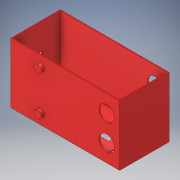
# Autodesk Inventor part: Torse
Saved by Autodesk Inventor 2019 (Build 230136000, 136)
## iProperties
Created: 2020-01-16
Part Number: Torse
Material: Générique
Document SubType Name: Modeling
Designer: Quentin
Density: 1 g/cm^3
Appearance: Rouge clair
Author: Quentin
Autodesk Inventor part; units mm, degrees
ref_plane "YZ Plane" through (0, 0, 0) normal (1, 0, 0) x (0, 1, 0)
ref_plane "XZ Plane" through (0, 0, 0) normal (0, 1, 0) x (-1, 0, 0)
ref_plane "XY Plane" through (0, 0, 0) normal (0, 0, 1) x (1, 0, 0)
sketch "Esquisse1" plane through (0, 0, 0) normal (1, 0, 0) x (0, 1, 0)
  line L0 (0, 0) -> (60, 0)
  line L1 (60, 0) -> (60, -50)
  line L2 (60, -50) -> (0, -50)
  line L3 (0, -50) -> (0, 0)
  dimension "d0" = 60
  dimension "d1" = 50
  constraints: 8 end point, 2 parallel, 1 horizontal, 1 perpendicular
  measures "d0" distance of L1.end L2.end
  measures "d1" distance of L0.end L1.end
extrude "Extrusion1" add sketch "Esquisse1" along normal blind 110
shell "Coque1" thickness 1 removed faces 1 at (36.6667, 0, -33.3333)
sketch "Esquisse2" plane through (0, 0, -50) normal (0, -1, 0) x (1, 0, 0)
  line L0 (0, 50) -> (110, 50) projected
  line L1 (110, 0) -> (110, 50) projected
  line L2 (110, 50) -> (110, 0)
  line L3 (110, 25) -> (110, 19)
  line L4 (110, 25) -> (110, 31)
  line L5 (0, 50) -> (0, 0) projected
  line L6 (84, 19) -> (61.25, 19)
  line L7 (84, 31) -> (61.25, 31)
  line L8 (110, 50) -> (0, 50)
  line L9 (0, 50) -> (0, 0)
  line L10 (0, 0) -> (110, 0) projected
  line L11 (0, 0) -> (110, 0)
  line L12 (109, 49) -> (109, 1) projected
  line L13 (110, 31) -> (110, 19)
  line L14 (110, 50) -> (110, 0) projected
  line L15 (61.25, 31) -> (57.25, 31)
  line L16 (57.25, 31) -> (57.25, 19)
  line L17 (82.25, 19) -> (86.25, 19)
  line L18 (109, 31) -> (105, 31)
  line L19 (80, 31) -> (80, 19)
  line L20 (1, 49) -> (109, 49) projected
  line L21 (57.25, 19) -> (61.25, 19)
  line L22 (110, 50) -> (80, 50)
  line L23 (0, 50) -> (110, 50) projected
  line L24 (80, 31) -> (80, 50)
  dimension "d5" = 6
  dimension "d6" = 6
  dimension "d7" = 48.75
  dimension "d50" = 4
  dimension "d67" = 30
  constraints: 34 end point, 6 perpendicular, 5 point on line, 3 collinear, 3 horizontal, 1 midpoint
  measures "d5" distance of L3.start L3.end
  measures "d6" distance of L3.start L4.end
  measures "d7" distance of L7.end L4.end
  measures "d50" distance of L18.start L18.end
  measures "d67" distance of L0.end L22.end
extrude "Extrusion2" add sketch "Esquisse2" along normal blind 1
sketch "Esquisse3" plane through (0, 0, 0) normal (-1, 0, 0) x (0, 0, 1)
  line L0 (0, 0) -> (-19, 0)
  line L1 (-19, 0) -> (-19, 10)
  line L2 (-19, 10) -> (-31, 10)
  line L3 (-31, 10) -> (-31, 33.75)
  line L4 (-31, 33.75) -> (-19, 33.75)
  line L5 (-19, 33.75) -> (-19, 10)
  dimension "d10" = 10
  dimension "d11" = 12
  dimension "d12" = 23.75
  constraints: 12 end point, 3 perpendicular, 2 horizontal, 1 collinear
  measures "d10" distance of L0.end L1.end
  measures "d11" distance of L1.end L2.end
  measures "d12" distance of L2.end L3.end
extrude "Extrusion3" cut sketch "Esquisse3" against normal blind 1
sketch "Esquisse4" plane through (110, 60, -50) normal (0, 0, -1) x (-1, 0, 0)
  line L0 (110, -61) -> (110, 0) projected
  line L1 (110, -61) -> (100, -61)
  line L2 (0, -61) -> (110, -61) projected
  line L3 (110, 0) -> (0, 0) projected
  circle A0 centre (80, -50.5) radius 4
  line L4 (110, 0) -> (0, 0) projected
  circle A1 centre (80, -10.5) radius 4
  line L5 (110, 0) -> (80, 0)
  line L6 (80, -10.5) -> (80, -50.5)
  line L7 (80, -50.5) -> (80, -61)
  point P0 (110, -60)
  dimension "d15" = 10
  dimension "d28" = 8
  dimension "d48" = 8
  dimension "d65" = 30
  dimension "d69" = 40
  dimension "d70" = 10.5
  constraints: 8 end point, 3 point on line, 2 centre point, 1 perpendicular, 1 vertical
  measures "d15" distance of L0.start L1.end
  measures "d28" diameter of A0
  measures "d48" diameter of A1
  measures "d65" distance of L0.end L5.end
  measures "d69" distance of L6.start L6.end
  measures "d70" distance of L6.end L7.end
extrude "Extrusion4" add sketch "Esquisse4" along normal blind 3
sketch "Esquisse8" plane through (0, 60, 0) normal (0, 0, 1) x (1, 0, 0)
  circle A0 centre (30, -10.5) radius 4
  line L0 (110, -61) -> (0, -61) projected
  circle A1 centre (30, -50.5) radius 4 projected
  circle A2 centre (30, -50.5) radius 4
  line L1 (30, -21.5) -> (30, -14.5)
  line L2 (30, -44.5) -> (30, -46.5)
  line L3 (0, -61) -> (0, 0) projected
  line L4 (0, 0) -> (30, 0)
  line L5 (0, 0) -> (110, 0) projected
  line L6 (30, -50.5) -> (30, -10.5)
  line L7 (1, -1) -> (109, -1) projected
  line L8 (30, -10.5) -> (30, 0)
  line L9 (30, -50.5) -> (30, -61)
  point P0 (0, -60)
  point P1 (30, -6.5)
  dimension "d74" = 8
  dimension "d40" = 8
  dimension "d66" = 30
  dimension "d73" = 40
  constraints: 12 end point, 3 point on line, 2 point on circle, 2 vertical, 1 centre point, 1 coincident, 1 vertical alignment, 2 other
  measures "d40" diameter of A0
  measures "d66" distance of L3.end L4.end
  measures "d73" distance of L6.start L6.end
extrude "Extrusion8" add sketch "Esquisse8" along normal blind 3 contours L6 L8 A0 | A0 L8 L6 | L6 L9 A1 | A1 L9 L6
sketch "Esquisse6" plane through (0, 60, 0) normal (0, 1, 0) x (1, 0, 0)
  line L0 (1, 49) -> (109, 49) projected
  line L1 (1, 1) -> (1, 49)
  line L2 (1, 49) -> (109, 49)
  line L3 (109, 49) -> (109, 1)
  line L4 (109, 1) -> (1, 1)
  line L5 (110, 0) -> (0, 0) projected
  constraints: 8 end point, 1 collinear, 1 parallel, 1 perpendicular, 1 vertical
extrude "Extrusion6" cut sketch "Esquisse6" against normal blind 10
sketch "Esquisse12" plane through (0, 60, 0) normal (0, 0, 1) x (1, 0, 0)
  line L0 (110, 0) -> (110, -61) projected
  line L1 (110, 0) -> (97, 0)
  line L2 (1, 0) -> (109, 0) projected
  line L3 (97, 0) -> (97, -17.5)
  circle A0 centre (97, -17.5) radius 7.8
  line L4 (97, -17.5) -> (97, -43.5)
  circle A1 centre (97, -43.5) radius 7.8
  point P0 (0, -60)
  dimension "d51" = 13
  dimension "d52" = 17.5
  dimension "d53" = 15.6
  dimension "d54" = 26
  dimension "d55" = 15.6
  constraints: 6 end point, 2 centre point, 2 coincident, 2 vertical, 1 point on line
  measures "d51" distance of L0.start L1.end
  measures "d52" distance of L1.end L3.end
  measures "d53" diameter of A0
  measures "d54" distance of L4.start L4.end
  measures "d55" diameter of A1
extrude "Extrusion9" cut sketch "Esquisse12" against normal through all
sketch "Esquisse13" plane through (0, -1, -50) normal (0, -1, 0) x (1, 0, 0)
  line L0 (0, 0) -> (110, 0) projected
  line L1 (110, 0) -> (97, 0)
  line L2 (97, 0) -> (97, 12)
  line L3 (97, 12) -> (97, 38)
  line L4 (97, 38) -> (97, 50)
  circle A0 centre (97, 38) radius 7.85
  circle A1 centre (97, 12) radius 7.85
  point P0 (0, 50)
  dimension "d58" = 13
  dimension "d59" = 12
  dimension "d60" = 26
  dimension "d61" = 15.7
  dimension "d62" = 15.7
  constraints: 8 end point, 2 centre point, 2 coincident, 2 point on line, 1 perpendicular, 1 vertical
  measures "d58" distance of L0.end L1.end
  measures "d59" distance of L1.end L2.end
  measures "d60" distance of L2.end L3.end
  measures "d61" diameter of A0
  measures "d62" diameter of A1
extrude "Extrusion10" cut sketch "Esquisse13" against normal blind 10
